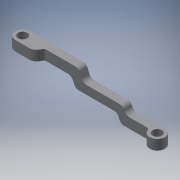
# Autodesk Inventor part: HbFingerMainCouplerLink01
Saved by Autodesk Inventor 2017 (Build 210142000, 142)
## iProperties
Created: 2015-02-23
Part Number: HbFingerMainCouplerLink01
Material: 一般
Document SubType Name: Modeling
Designer: Yamaura
Density: 1 g/cm^3
Appearance: 既定
Author: Yamaura
Autodesk Inventor part; units mm, degrees
ref_plane "YZ Plane" through (0, 0, 0) normal (1, 0, 0) x (0, 1, 0)
ref_plane "XZ Plane" through (0, 0, 0) normal (0, 1, 0) x (-1, 0, 0)
ref_plane "XY Plane" through (0, 0, 0) normal (0, 0, 1) x (1, 0, 0)
sketch "スケッチ1" plane through (0, 0, 0) normal (0, 0, 1) x (1, 0, 0)
  circle A0 centre (0, 0) radius 1.7
  circle A1 centre (48, 0) radius 1.7
  circle A2 centre (0, 0) radius 3
  circle A3 centre (48, 0) radius 3
  line L0 (0, 3) -> (48, 3)
  line L1 (0, -3) -> (48, -3)
  dimension "d0" = 3.4
  dimension "d1" = 3.4
  dimension "d2" = 6
  dimension "d3" = 6
  dimension "d4" = 48
  constraints: 4 centre point, 4 end point, 4 point on circle, 4 tangent, 3 coincident, 1 horizontal alignment
  measures "d0" diameter of A0
  measures "d1" diameter of A1
  measures "d2" diameter of A2
  measures "d3" diameter of A3
  measures "d4" distance of A1.centre point (0, 0)
extrude "押し出し1" add sketch "スケッチ1" along normal mid plane 4
offset faces "サイズ1" outward -0.05 faces at (49.6945, -0.1368, 0.6667)
offset faces "サイズ2" outward -0.05 faces at (1.6945, 0.1368, -0.6667)
scale "尺度1" factors (0.8836555, 0.8836555, 0.8836555) then translate (2.7923, 0.349, -0.2327) bodies 1
sketch "スケッチ2" plane through (2.7923, -2.3019, 1.5346) normal (0, 0, 1) x (1, 0, 0)
  circle A0 centre (0, 2.651) radius 1.5464 projected
  circle A1 centre (0, 2.651) radius 1.65
  circle A2 centre (42.4155, 2.651) radius 1.5464 projected
  circle A3 centre (42.4155, 2.651) radius 1.65
  point P0 (-2.7923, 2.3019)
  dimension "d12" = 3.3
  constraints: 2 centre point, 2 coincident, 1 equal radius
  measures "d12" diameter of A1
extrude "押し出し2" cut sketch "スケッチ2" against normal up to next
sketch "スケッチ3" plane through (2.7923, -2.3019, 1.5346) normal (0, 0, 1) x (1, 0, 0)
  circle A0 centre (0, 2.651) radius 1.65 projected
  circle A1 centre (42.4155, 2.651) radius 1.65 projected
  arc A2 (0, 5.3019) -> (0, 0) centre (0, 2.651) ccw projected
  line L0 (0, 0) -> (42.4155, 0) projected
  arc A3 (42.4155, 0) -> (42.4155, 5.3019) centre (42.4155, 2.651) ccw projected
  line L1 (42.4155, 5.3019) -> (0, 5.3019) projected
  point P0 (-2.7923, 2.3019)
extrude "押し出し3" add sketch "スケッチ3" along normal blind 6
sketch "スケッチ4" plane through (2.7923, 3, -2) normal (0, 1, 0) x (1, 0, 0)
  line L0 (42.4155, -9.5346) -> (45.0664, -9.5346) projected
  line L1 (45.0664, -9.5346) -> (45.0664, -3.5346)
  line L2 (45.0664, 0) -> (45.0664, -9.5346) projected
  line L3 (45.0664, -3.5346) -> (17.4176, -3.5346)
  line L4 (-2.651, 0) -> (-2.651, -6)
  line L5 (-2.651, 0) -> (-2.651, -9.5346) projected
  line L6 (-2.651, -6) -> (12.349, -6)
  line L7 (12.349, -6) -> (15.0664, 0)
  line L8 (42.4155, 0) -> (0, 0) projected
  line L9 (15.0664, 0) -> (-2.651, 0)
  line L10 (17.4176, -3.5346) -> (14.7002, -9.5346)
  line L11 (14.7002, -9.5346) -> (45.0664, -9.5346)
  line L12 (42.4155, -9.5346) -> (0, -9.5346) projected
  line L13 (0, 0) -> (42.4155, 0) projected
  point P0 (-2.7923, -2)
  dimension "d17" = 6
  dimension "d18" = 6
  dimension "d20" = 3.6
  dimension "d21" = 30
  dimension "d22" = 15
  constraints: 16 end point, 3 parallel, 3 point on line, 2 horizontal, 2 perpendicular
  measures "d17" distance between parallel lines of L9 L6
  measures "d18" distance between parallel lines of L3 L12
  measures "d20" distance between parallel lines of L7 L10
  measures "d21" distance from line of L2 L7.end
  measures "d22" distance of L4.end L6.end
extrude "押し出し4" cut sketch "スケッチ4" against normal through all
sketch "スケッチ5" plane through (2.7923, -2.3019, 7.5346) normal (0, 0, 1) x (1, 0, 0)
  circle A0 centre (0, 2.651) radius 1.65 projected
  line L0 (0, 0) -> (14.7002, 0) projected
  arc A1 (0, 0) -> (2.6467, 2.5) centre (0, 2.651) ccw
  line L1 (2.6467, 2.5) -> (39.7688, 2.5)
  line L2 (0, 0) -> (42.4155, 0)
  line L3 (42.4155, 0) -> (15.0664, 0) projected
  arc A2 (39.7688, 2.5) -> (42.4155, 0) centre (42.4155, 2.651) ccw
  point P0 (-2.7923, 2.3019)
  dimension "d28" = 2.5
  constraints: 4 end point, 4 point on circle, 2 centre point, 2 coincident, 1 horizontal, 1 point on line, 1 tangent
  measures "d28" distance between parallel lines of L2 L1
extrude "押し出し5" cut sketch "スケッチ5" against normal up to next contours A1 L1 A2 L2 L0
fillet "フィレット1" radius 1 2 edges at (42.5611, 0.1981, -0.2327) (5.4389, 0.1981, 5.7673)
sketch "スケッチ6" plane through (2.7923, -2.3019, 7.5346) normal (0, 0, 1) x (1, 0, 0)
  circle A0 centre (-5, 2.651) radius 1.65
  circle A1 centre (-5, 2.651) radius 2.651
  arc A2 (0, 5.3019) -> (2.5158, 1.8152) centre (0, 2.651) ccw projected
  circle A3 centre (0, 2.651) radius 1.65 projected
  line L0 (-5, 0) -> (0, 0)
  arc A4 (0, 5.3019) -> (2.5158, 1.8152) centre (0, 2.651) ccw projected
  line L1 (12.349, 5.3019) -> (0, 5.3019) projected
  line L2 (-5, 5.3019) -> (0, 5.3019)
  arc A5 (0, 0) -> (0, 5.3019) centre (0, 2.651) ccw
  point P0 (-2.7923, 2.3019)
  dimension "d32" = 5
  constraints: 6 point on circle, 4 end point, 3 centre point, 2 coincident, 2 equal radius, 2 tangent, 1 collinear, 1 horizontal alignment
  measures "d32" distance of A0.centre A2.centre
extrude "押し出し6" add sketch "スケッチ6" against normal up to surface (3.5346 mm away) contours A1 A2 | L2 A2 A1 | A1 A2 L0 | A2 A5 A1 | A1 A2 | A3
fillet "フィレット2" radius 2 2 edges at (20.2099, 1.599, 1.5346) (15.1413, 1.599, 4)
sketch "スケッチ7" plane through (17.8587, 3, -2) normal (0, 1, 0) x (1, 0, 0)
  line L0 (-0.3662, -9.5346) -> (1.8191, -4.7095) projected
  line L1 (1.3095, -5.8346) -> (15.3095, -5.8346)
  line L2 (15.3095, -5.8346) -> (16.3512, -3.5346)
  line L3 (3.6409, -3.5346) -> (23.8842, -3.5346) projected
  line L4 (16.3512, -3.5346) -> (2.3512, -3.5346)
  line L5 (2.3512, -3.5346) -> (1.3095, -5.8346)
  line L6 (-0.3662, -9.5346) -> (1.8191, -4.7095) projected
  point P0 (-17.8587, -2)
  dimension "d36" = 2.3
  dimension "d37" = 14
  constraints: 8 end point, 2 horizontal, 2 point on line, 1 collinear, 1 parallel
  measures "d36" distance between parallel lines of L4 L1
  measures "d37" distance of L1.start L1.end
extrude "押し出し7" add sketch "スケッチ7" against normal up to surface (2.8019 mm away)
fillet "フィレット3" radius 2 2 edges at (19.1682, 1.599, 3.8346) (34.2099, 1.599, 1.5346)
sketch "スケッチ8" plane through (17.8587, 3, -2) normal (0, 1, 0) x (1, 0, 0)
  line L0 (0, 0) -> (27.349, 0) projected
  line L1 (14.6587, 0) -> (13.3749, -2.8346)
  line L2 (13.3749, -2.8346) -> (-1.2838, -2.8346)
  line L3 (0, 0) -> (-2.1853, -4.8251) construction
  line L4 (-1.2838, -2.8346) -> (0, 0)
  line L5 (0, 0) -> (14.6587, 0)
  line L6 (2.5993, -5.8346) -> (15.3095, -5.8346) projected
  line L7 (15.3095, -5.8346) -> (15.8191, -4.7095) projected
  point P0 (-17.8587, -2)
  dimension "d41" = 3
  dimension "d42" = 3
  constraints: 8 end point, 2 parallel, 2 point on line, 1 horizontal
  measures "d41" distance between parallel lines of L6 L2
  measures "d42" distance between parallel lines of L7 L1
extrude "押し出し8" cut sketch "スケッチ8" against normal through all
fillet "フィレット4" radius 1.5 5 edges at (16.5749, 1.599, 0.8346) (31.2336, 1.599, 0.8346) (32.5174, 1.599, -2) (17.4925, 1.599, 7.5346) (33.1682, 1.599, 3.8346)
